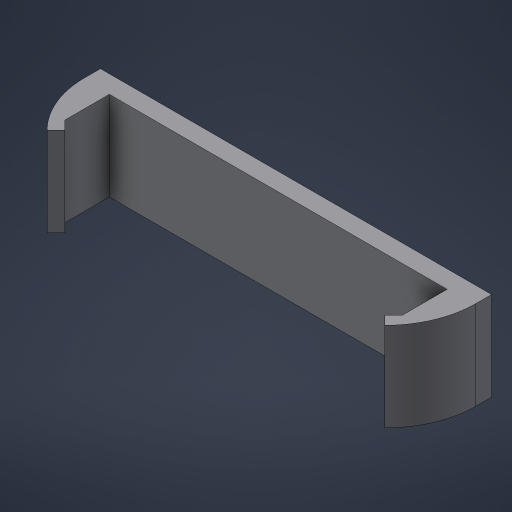
# Autodesk Inventor part: TrackIR
Saved by Autodesk Inventor 2023.5 (Build 275446000, 446)
## iProperties
Created: 2025-03-20
Part Number: TrackIR
Material: Generisch
Document SubType Name: Modeling
Designer: David Lill
Density: 1 g/cm^3
Appearance: Vorgabe
Author: David Lill
## iProperties of the stored document TrackIR_3D-Druck.ipt
Part Number: TrackIR_3D-Druck
Material: Allgemein
Document SubType Name: Modellieren
Designer: David Lill
Appearance: Vorgabe
Author: David Lill
Autodesk Inventor part; units mm, degrees
ref_plane "YZ Plane" through (0, 0, 0) normal (1, 0, 0) x (0, 1, 0)
ref_plane "XZ Plane" through (0, 0, 0) normal (0, 1, 0) x (-1, 0, 0)
ref_plane "XY Plane" through (0, 0, 0) normal (0, 0, 1) x (1, 0, 0)
sketch "Skizze1" plane through (0, 0, 0) normal (0, 0, 1) x (1, 0, 0)
  line L0 (0, 0) -> (-19, 0)
  line L1 (-19, 0) -> (-19, -5)
  line L2 (-19, -5) -> (-18, -6)
  line L3 (-18, -6) -> (-19, -7)
  arc A0 (-22, 0.2426) -> (-19, -7) centre (-11.7574, 0.2426) ccw
  line L4 (-22, 0.2426) -> (-22, 2)
  line L5 (-22, 2) -> (0, 2)
  line L6 (0, 2) -> (0, 0)
  dimension "d6" = 19
  dimension "d7" = 5
  dimension "d8" = 3
  dimension "d9" = 1
  dimension "d10" = 2
  dimension "d11" = 2
  constraints: 14 end point, 3 perpendicular, 2 point on circle, 2 point on line, 2 vertical, 1 centre point, 1 horizontal, 1 tangent, 1 vertical alignment
  measures "d6" distance of L0.start L0.end
  measures "d7" distance of L0.end L1.end
  measures "d8" distance between parallel lines of L4 L1
  measures "d9" distance from line of L1 L2.end
  measures "d10" distance of L3.end L1.end
  measures "d11" distance between parallel lines of L0 L5
extrude "Extrusion1" add sketch "Skizze1" along normal blind 10
mirror "Spiegeln1" about plane through (0, 0, 0) normal (1, 0, 0) of "Extrusion1"
